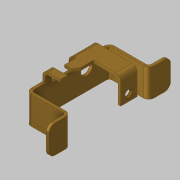
# Autodesk Inventor part: Part_final
Saved by Autodesk Inventor 2019 (Build 230136000, 136)
## iProperties
Created: 2019-05-20
Part Number: Part_final
Material: Brass, Soft Yellow
Document SubType Name: Sheet Metal
Designer: Emily Rojas
Density: 8.47 g/cm^3
Sheet Metal Rule: Default
Appearance: Brass - Satin
Flat Pattern Width: 11.4572 cm
Flat Pattern Length: 22.0143 cm
Flat Pattern Area: 252.222 cm^2
Sheet Metal Width: 114,572 mm
Sheet Metal Length: 220,143 mm
Sheet Metal Area: 25222,195 mm^2
Author: Emily Rojas
Autodesk Inventor part; units mm, degrees
ref_plane "YZ Plane" through (0, 0, 0) normal (1, 0, 0) x (0, 1, 0)
sketch "Sketch1" plane through (0, 0, 0) normal (0, 1, 0) x (-1, 0, 0)
  line L0 (0, 0) -> (0, -22)
  line L1 (0, -22) -> (45, -22)
  line L2 (45, -22) -> (45, -117)
  line L3 (45, -117) -> (0, -117)
  line L4 (0, -117) -> (0, -139)
  dimension "d0" = 22
  dimension "d1" = 45
  dimension "d2" = 22
  dimension "d3" = 95
  measures "d0" distance from line of L4.end L3
  measures "d1" distance from line of L2 L3.end
  measures "d2" distance from line of L0.start L1
  measures "d3" distance between parallel lines of L1 L3
contour flange "Contour Flange1" sketch "Sketch1" thickness 3 bend radius 3 width 32 along (0, 1, 0) mid plane no both sides no wall seen from (0, 0, -11) lies toward (1, 0, 0) curves L0 L1 L2 L3 L4
bend "Bend1"
corner "Corner1"
fillet "Corner Round1" radius 7 4 edges at (1.5, 32, -139) (1.5, 0, -139) (1.5, 32, 0) (1.5, 0, 0)
sketch "Sketch2" plane through (-45, 0, -111) normal (-1, 0, 0) x (0, 0, 1)
  line L0 (83, 0) -> (0, 0) projected
  line L1 (-3, 32) -> (-3, 0) projected
  line L2 (-6, 0) -> (-6, 32) projected
  point P0 (111, 0)
  point P1 (23, 22)
  dimension "d23" = 22
  dimension "d68" = 29
  measures "d23" distance from line of L0 point (23, 22)
  measures "d68" distance from line of L2 point (23, 22)
hole "Hole1" at (-45, 22, -88) direction (1, 0, 0) diameter 13 end through all
ref_plane "Work Plane1" through (-39, 0, -41) normal (0, 0, 1) x (1, 0, 0)
sketch "Sketch5" plane through (-39, 0, -41) normal (0, 0, 1) x (1, 0, 0)
  line L0 (-6, 32) -> (-6, 44)
  line L1 (-6, 44) -> (14, 44)
  point P0 (39, 0)
  dimension "d26" = 12
  dimension "d27" = 20
  measures "d26" distance of L0.start L0.end
  measures "d27" distance of L0.end L1.end
contour flange "Contour Flange2" sketch "Sketch5" thickness 3 bend radius 3 width 8 along (0, 0, -1) mid plane no both sides no wall seen from (-45, 38, -41) lies toward (1, 0, 0) curves L0 L1
bend "Bend2"
corner "Corner2"
ref_plane "Work Plane2" through (-39, 0, -71) normal (0, 0, 1) x (1, 0, 0)
sketch "Sketch6" plane through (-39, 0, -71) normal (0, 0, 1) x (1, 0, 0)
  line L0 (-6, 32) -> (-6, 44)
  line L1 (-6, 44) -> (45, 44)
  line L2 (45, 44) -> (45, 14)
  point P0 (39, 0)
  dimension "d39" = 12
  dimension "d41" = 51
  dimension "d42" = 30
  measures "d39" distance of L0.start L0.end
  measures "d41" distance of L0.end L1.end
  measures "d42" distance of L1.end L2.end
contour flange "Contour Flange3" sketch "Sketch6" thickness 3 bend radius 3 width 27 along (0, 0, -1) mid plane no both sides no wall seen from (-45, 38, -71) lies toward (1, 0, 0) curves L0 L1 L2
bend "Bend3"
corner "Corner3"
sketch "Sketch7" plane through (3, 14, -98) normal (-1, 0, 0) x (0, 0, 1)
  line L0 (70, -14) -> (-13, -14) projected
  line L1 (-16, 18) -> (-16, -14) projected
  line L2 (-19, -14) -> (-19, 18) projected
  point P0 (98, -14)
  point P1 (10, 8)
  dimension "d69" = 29
  dimension "d70" = 22
  measures "d69" distance from line of L2 point (10, 8)
  measures "d70" distance from line of L0 point (10, 8)
hole "Hole2" at (3, 22, -88) direction (1, 0, 0) diameter 8 end through all
sketch "Sketch8" plane through (-39, 44, -98) normal (0, 1, 0) x (1, 0, 0)
  line L0 (14, -19) -> (51.8271, -19)
  line L1 (51.8271, -19) -> (51.8271, -35.7811)
  line L2 (51.8271, -35.7811) -> (14, -35.7811)
  line L3 (14, -35.7811) -> (14, -19)
  line L4 (-6, 0) -> (-6, -27) projected
  line L5 (0, 0) -> (39, 0) projected
  point P0 (39, -98)
  dimension "d62" = 20
  dimension "d63" = 19
  constraints: 8 end point, 2 parallel, 1 horizontal, 1 perpendicular
  measures "d62" distance between parallel lines of L4 L3
  measures "d63" distance between parallel lines of L5 L0
extrude "Extrusion1" cut sketch "Sketch8" against normal through all
sketch "Sketch9" plane through (-45, 32, -49) normal (0, 1, 0) x (1, 0, 0)
  line L0 (0, 0) -> (3, 0) projected
  line L1 (3, 0) -> (3, 22) projected
  line L2 (0, 0) -> (3, 0)
  line L3 (3, 0) -> (3, 22)
  line L4 (3, 22) -> (0, 22)
  line L5 (0, 22) -> (0, 0)
  point P0 (45, -49)
  constraints: 8 end point, 2 parallel, 1 horizontal, 1 perpendicular
extrude "Extrusion2" cut sketch "Sketch9" against normal blind 3.5
sketch "Sketch10" plane through (-39, 41, -71) normal (0, 0, 1) x (1, 0, 0)
  line L0 (14, 0) -> (14, 3) projected
  line L1 (0, 3) -> (14, 3) projected
  line L2 (14, 0) -> (2, 0)
  line L3 (2, 0) -> (2, 3)
  line L4 (2, 3) -> (14, 3)
  line L5 (14, 3) -> (14, 0)
  point P0 (39, -41)
  dimension "d71" = 12
  constraints: 8 end point, 2 parallel, 1 horizontal, 1 perpendicular, 1 point on line
  measures "d71" distance between parallel lines of L3 L0
extrude "Extrusion3" add sketch "Sketch10" along normal blind 13
chamfer "Corner Chamfer1" distance 4 distance2 6 1 edges at (-25, 42.5, -58) measured on face at (-25.5, 42.5, -58)
equation "\"d21\" = Thickness"
equation "\"d58\" = Thickness"
equation "\"d4\" = Thickness"
equation "\"d5\" = BendReliefWidth"
equation "\"d6\" = BendReliefDepth"
equation "\"d7\" = MinimumRemnant"
equation "\"d8\" = TransitionRadius"
equation "\"d10\" = BendRadius"
equation "\"d12\" = CornerReliefSize"
equation "\"d13\" = GapSize"
equation "\"d14\" = JacobiRadiusSize"
equation "\"d28\" = BendReliefWidth"
equation "\"d29\" = BendReliefDepth"
equation "\"d30\" = MinimumRemnant"
equation "\"d31\" = TransitionRadius"
equation "\"d33\" = BendRadius"
equation "\"d35\" = CornerReliefSize"
equation "\"d36\" = GapSize"
equation "\"d37\" = JacobiRadiusSize"
equation "\"d43\" = BendReliefWidth"
equation "\"d44\" = BendReliefDepth"
equation "\"d45\" = MinimumRemnant"
equation "\"d46\" = TransitionRadius"
equation "\"d48\" = BendRadius"
equation "\"d50\" = CornerReliefSize"
equation "\"d51\" = GapSize"
equation "\"d52\" = JacobiRadiusSize"
equation "\"BendRadius\" = Thickness"
equation "\"BendReliefWidth\" = Thickness"
equation "\"BendReliefDepth\" = 0.5 * Thickness"
equation "\"CornerReliefSize\" = 4 * Thickness"
equation "\"MinimumRemnant\" = 2 * Thickness"
equation "\"TransitionRadius\" = BendRadius"
equation "\"JacobiRadiusSize\" = Thickness"
equation "\"GapSize\" = Thickness"
equation "\"Thickness\" = 3"
body "Solid1"
